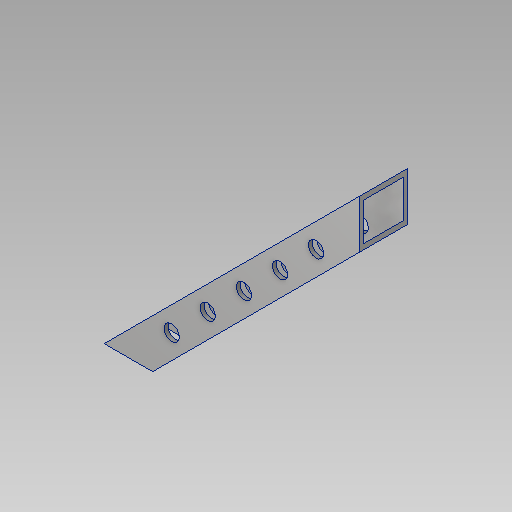
# Autodesk Inventor part: C002
Saved by Autodesk Inventor 2017 (Build 210142000, 142)
## iProperties
Created: 2017-06-13
Part Number: C002
Material: Aluminum 6061
Document SubType Name: Modeling
Designer: zallen
Density: 2.7 g/cm^3
Appearance: Aluminum - Flat
Mass: 30.515 g
Surface Area: 153.189 cm^2
Volume: 11.3018 cm^3
Author: zallen
Autodesk Inventor part; units mm, degrees
ref_plane "YZ Plane" through (0, 0, 0) normal (1, 0, 0) x (0, 1, 0)
ref_plane "XZ Plane" through (0, 0, 0) normal (0, 1, 0) x (-1, 0, 0)
ref_plane "XY Plane" through (0, 0, 0) normal (0, 0, 1) x (1, 0, 0)
sketch "Sketch1" plane through (0, 0, 0) normal (0, 0, 1) x (1, 0, 0)
  line L0 (0, 0) -> (100, 0) construction
  line L1 (100, 0) -> (100, 100) construction
  line L2 (100, 100) -> (0, 100) construction
  line L3 (0, 100) -> (0, 0) construction
  line L4 (0, 0) -> (100, 100)
  line L5 (0, 0) -> (19, 0)
  line L6 (100, 100) -> (100, 81)
  line L7 (19, 0) -> (100, 81)
  dimension "d1" = 100
  dimension "d2" = 100
  dimension "d3" = 19
  dimension "d4" = 19
  constraints: 16 end point, 2 parallel, 2 point on line, 1 horizontal, 1 perpendicular
  measures "d1" distance of L2.end L1.end
  measures "d2" distance of L1.end L0.end
  measures "d3" distance of L0.start L5.end
  measures "d4" distance of L1.end L6.end
extrude "Extrusion1" add sketch "Sketch1" along normal blind 19
ref_plane "Work Plane1" through (59.5, 40.5, 19) normal (-0.7071068, -0.7071068, 0) x (-0.7071068, 0.7071068, 0)
sketch "Sketch2" plane through (59.5, 40.5, 19) normal (-0.7071068, -0.7071068, 0) x (-0.7071068, 0.7071068, 0)
  line L0 (13.435, 19) -> (0, 19) projected
  line L1 (13.435, 19) -> (13.435, 0) projected
  line L2 (0, 0) -> (13.435, 0) projected
  line L3 (0, 19) -> (0, 0) projected
  line L4 (11.935, 1.5) -> (11.935, 17.5)
  line L5 (11.935, 17.5) -> (1.5, 17.5)
  line L6 (1.5, 17.5) -> (1.5, 1.5)
  line L7 (1.5, 1.5) -> (11.935, 1.5)
  point P0 (13.435, 19)
  dimension "d7" = 1.5
  constraints: 8 end point, 3 other
  measures "d7" distance between parallel lines of L2 L7
extrude "Extrusion2" cut sketch "Sketch2" along normal through all both and the other way through all contours L7 L6 L5 L4
sketch "Sketch3" plane through (0, 0, 19) normal (0, 0, 1) x (1, 0, 0)
  line L0 (19, 0) -> (0, 0) construction
  line L1 (100, 97.8787) -> (100, 83.1213) construction
  circle A0 centre (26.4657, 16.9657) radius 3
  circle A1 centre (40.6079, 31.1079) radius 3
  circle A2 centre (54.75, 45.25) radius 3
  circle A3 centre (83.0343, 73.5343) radius 3
  circle A4 centre (68.8921, 59.3921) radius 3
  line L2 (26.4657, 16.9657) -> (83.0343, 73.5343) construction
  line L3 (100, 81) -> (19, 0) projected
  line L4 (59.5, 40.5) -> (50, 50) construction
  line L5 (100, 100) -> (0, 0) projected
  line L6 (9.5, 0) -> (100, 90.5) construction
  point P0 (54.75, 45.25)
  dimension "d10" = 6
  dimension "d12" = 6
  dimension "d13" = 20
  dimension "d14" = 6
  dimension "d15" = 6
  dimension "d16" = 6
  dimension "d17" = 20
  dimension "d18" = 20
  dimension "d19" = 20
  constraints: 7 midpoint, 6 end point, 5 centre point
  measures "d10" diameter of A0
  measures "d12" diameter of A1
  measures "d13" distance of A1.centre L2.start
  measures "d14" diameter of A2
  measures "d15" diameter of A3
  measures "d16" diameter of A4
  measures "d17" distance of A2.centre A1.centre
  measures "d18" distance of A2.centre A4.centre
  measures "d19" distance of L2.end A4.centre
extrude "Extrusion3" cut sketch "Sketch3" against normal through all
body "Solid1"
